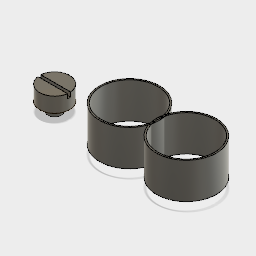
upper stand and glasses v1 (Autodesk Fusion 360 design; units mm, degrees)
Autodesk Fusion 360 part; units mm, degrees
sketch "Sketch1" plane through (0, 0, 0) normal (0, 1, 0) x (1, 0, 0)
cylinder "CylinderPrimitive1" add diameter 10 height 5 placed x (1, 0, 0) y (0, 0, -1) z (0, 1, 0) at (0, 0, 0) makes body 1
sketch "Sketch2" plane through (0, 0, 0) normal (0, -1, 0) x (1, 0, 0)
  circle A0 centre (0, 0) radius 5
cylinder "CylinderPrimitive2" add diameter 4.5 height 3 placed x (1, 0, 0) y (0, 0, 1) z (0, -1, 0) at (0, 0, 0) bodies 1
box "BoxPrimitive1" cut length 1 width 13 height -1.5 placed x (0, 0, -1) y (-1, 0, 0) z (0, 1, 0) at (7.0121, 5, 0.6528) bodies 1
sketch "Sketch4" plane through (0, 0, 0) normal (0, 1, 0) x (1, 0, 0)
  circle A0 centre (25, 0) radius 10
  circle A1 centre (25, 0) radius 9.5
  dimension "d10" = 20
  dimension "d11" = 0.5
  measures "d10" diameter of A0
extrude "Extrude1" add sketch "Sketch4" along normal blind 12 separate body makes body 2
copy_body "CopyPasteBodies1" bodies 2 makes body 3
move_body "Move1" bodies 3 to x (1, 0, 0) y (0, 1, 0) z (0, 0, 1) at (19, 0, 0)
